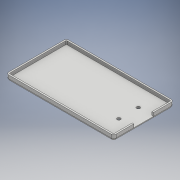
# Autodesk Inventor part: NodeLid
Saved by Autodesk Inventor 2018.3 (Build 223284000, 284)
## iProperties
Created: 2019-03-18
Part Number: NodeLid
Material: Generic
Document SubType Name: Modeling
Designer: matth
Density: 1 g/cm^3
Appearance: Default
Author: matth
Autodesk Inventor part; units mm, degrees
ref_plane "YZ Plane" through (0, 0, 0) normal (1, 0, 0) x (0, 1, 0)
ref_plane "XZ Plane" through (0, 0, 0) normal (0, 1, 0) x (-1, 0, 0)
ref_plane "XY Plane" through (0, 0, 0) normal (0, 0, 1) x (1, 0, 0)
sketch "Sketch1" plane through (0, 0, 0) normal (0, 0, 1) x (1, 0, 0)
  line L0 (-13.0469, 37.9774) -> (50.4531, 37.9774)
  line L1 (50.4531, 37.9774) -> (50.4531, 2.4174)
  line L2 (50.4531, 2.4174) -> (-13.0469, 2.4174)
  line L3 (-13.0469, 2.4174) -> (-13.0469, 37.9774)
  line L4 (49.5531, 37.0774) -> (-12.1469, 37.0774)
  line L5 (-12.1469, 37.0774) -> (-12.1469, 3.3174)
  line L6 (-12.1469, 3.3174) -> (49.5531, 3.3174)
  line L7 (49.5531, 3.3174) -> (49.5531, 37.0774)
  point P0 (0, 0)
  dimension "d0" = 63.5
  dimension "d1" = 35.56
  dimension "d2" = 0.9
  constraints: 16 end point, 4 parallel, 2 perpendicular, 1 horizontal, 3 other
  measures "d0" distance of L1.end L2.end
  measures "d1" distance of L2.end L0.start
  measures "d2" distance between parallel lines of L0 L4
extrude "Extrusion1" add sketch "Sketch1" along normal blind 2
sketch "Sketch2" plane through (0, 0, 0) normal (0, 0, -1) x (-1, 0, 0)
  line L0 (-50.4531, 2.4174) -> (13.0469, 2.4174) projected
  line L1 (13.0469, 2.4174) -> (13.0469, 37.9774) projected
  line L2 (13.0469, 37.9774) -> (-50.4531, 37.9774) projected
  line L3 (-50.4531, 37.9774) -> (-50.4531, 2.4174) projected
  point P0 (0, 0)
extrude "Extrusion2" add sketch "Sketch2" along normal blind 1
fillet "Fillet1" radius 1.5 4 edges at (-13.0469, 2.4174, 0.5) (50.4531, 2.4174, 0.5) (50.4531, 37.9774, 0.5) (-13.0469, 37.9774, 0.5)
fillet "Fillet2" radius 0.4 4 edges at (-12.1469, 37.0774, 1) (-12.1469, 3.3174, 1) (49.5531, 37.0774, 1) (49.5531, 3.3174, 1)
sketch "Sketch3" plane through (50.4531, 3.9174, 2) normal (1, 0, 0) x (0, 0, -1)
  line L0 (0, 32.56) -> (0, 0) projected
  line L1 (0, 10.5) -> (2, 10.5)
  line L2 (2, 10.5) -> (2, 22.06)
  line L3 (2, 22.06) -> (0, 22.06)
  line L4 (0, 22.06) -> (0, 10.5)
  line L5 (0, -1.5) -> (3, -1.5) projected
  line L6 (3, 34.06) -> (0, 34.06) projected
  point P0 (2, -3.9174)
  dimension "d9" = 2
  dimension "d10" = 12
  dimension "d11" = 12
  constraints: 8 end point, 2 parallel, 1 horizontal, 1 perpendicular, 1 point on line
  measures "d9" distance of L1.start L1.end
  measures "d10" distance between parallel lines of L5 L1
  measures "d11" distance between parallel lines of L6 L3
extrude "Extrusion3" cut sketch "Sketch3" against normal blind 1
chamfer "Chamfer1" distance 0.5 distance2 1 8 edges at (50.4531, 20.1974, -1) (50.0138, 2.8567, -1) (18.7031, 2.4174, -1) (-12.6075, 2.8567, -1) (-13.0469, 20.1974, -1) (-12.6075, 37.5381, -1) (18.7031, 37.9774, -1) (50.0138, 37.5381, -1) measured on face at (49.6602, 37.1845, -1) measured on face at (18.7031, 37.4774, -1) measured on face at (18.7031, 2.9174, -1) measured on face at (49.9531, 20.1974, -1) measured on face at (-12.254, 3.2103, -1) measured on face at (-12.5469, 20.1974, -1) measured on face at (-12.254, 37.1845, -1) measured on face at (49.6602, 3.2103, -1)
sketch "Sketch4" plane through (0, 0, -1) normal (0, 0, -1) x (-1, 0, 0)
  circle A0 centre (-41.4531, 25.9774) radius 1
  line L0 (11.5469, 37.9774) -> (-48.9531, 37.9774) projected
  line L1 (-50.4531, 36.4774) -> (-50.4531, 25.9774) projected
  circle A1 centre (-41.4531, 14.4174) radius 1
  line L2 (-48.9531, 2.4174) -> (11.5469, 2.4174) projected
  point P0 (0, 0)
  dimension "d17" = 2
  dimension "d18" = 12
  dimension "d19" = 9
  dimension "d22" = 2
  dimension "d23" = 12
  constraints: 2 centre point
  measures "d17" diameter of A0
  measures "d18" distance from line of L0 A0.centre
  measures "d19" distance from line of A0.centre L1
  measures "d22" diameter of A1
  measures "d23" distance from line of L2 A1.centre
extrude "Extrusion4" cut sketch "Sketch4" against normal blind 2
equation "\"d20\" = d22"
body "Solid1"
